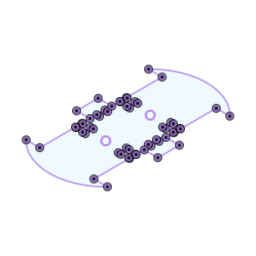
rover_M_v2_FF (Autodesk Fusion 360 design; units mm, degrees)
Autodesk Fusion 360 part; units mm, degrees
sketch "Sketch1" plane through (0, 0, 0) normal (0, 0, 1) x (1, 0, 0)
  line L0 (0, 0) -> (75, 0) construction
  line L1 (0, 0) -> (0, 145) construction
  line L2 (75, 0) -> (75, 20)
  line L3 (75, 20) -> (50, 20)
  line L4 (50, 20) -> (50, 113)
  line L5 (50, 113) -> (75, 113)
  arc A0 (75, 113) -> (0, 145) centre (0, 41.1094) ccw
  line L6 (0, 145) -> (-55.6559, 145) construction
  line L7 (-75, 0) -> (-75, 20)
  line L8 (-75, 20) -> (-50, 20)
  line L9 (-50, 20) -> (-50, 113)
  line L10 (-50, 113) -> (-75, 113)
  arc A1 (0, 145) -> (-75, 113) centre (0, 41.1094) ccw
  line L11 (75, 0) -> (75, -20)
  line L12 (75, -20) -> (50, -20)
  line L13 (50, -20) -> (50, -113)
  line L14 (50, -113) -> (75, -113)
  arc A2 (0, -145) -> (75, -113) centre (0, -41.1094) ccw
  line L15 (-50, -113) -> (-75, -113)
  line L16 (-50, -20) -> (-50, -113)
  line L17 (-75, -20) -> (-50, -20)
  line L18 (-75, 0) -> (-75, -20)
  arc A3 (-75, -113) -> (0, -145) centre (0, -41.1094) ccw
  line L19 (50, 35) -> (48.5, 35)
  line L20 (48.5, 35) -> (48.5, 47)
  line L21 (48.5, 47) -> (50, 47)
  line L22 (50, 47) -> (50, 35)
  line L23 (-50, 47) -> (-50, 35)
  line L24 (-50, 35) -> (-48.5, 35)
  line L25 (-48.5, 35) -> (-48.5, 47)
  line L26 (-48.5, 47) -> (-50, 47)
  line L27 (-48.5, -47) -> (-50, -47)
  line L28 (-50, -47) -> (-50, -35)
  line L29 (50, -47) -> (50, -35)
  line L30 (50, -35) -> (48.5, -35)
  line L31 (-50, -35) -> (-48.5, -35)
  line L32 (48.5, -35) -> (48.5, -47)
  line L33 (-48.5, -35) -> (-48.5, -47)
  line L34 (48.5, -47) -> (50, -47)
  line L35 (-50, 7.5) -> (-45, 7.5)
  line L36 (-45, 7.5) -> (-45, -7.5)
  line L37 (-45, -7.5) -> (-50, -7.5)
  line L38 (-50, -7.5) -> (-50, 7.5)
  line L39 (-45, 0) -> (0, 0) construction
  line L40 (50, 7.5) -> (45, 7.5)
  line L41 (45, 7.5) -> (45, -7.5)
  line L42 (45, -7.5) -> (50, -7.5)
  line L43 (50, -7.5) -> (50, 7.5)
  line L44 (-35.5, 48.5) -> (-30.5, 48.5)
  line L45 (-30.5, 48.5) -> (-30.5, 33.5)
  line L46 (-30.5, 33.5) -> (-35.5, 33.5)
  line L47 (-35.5, 33.5) -> (-35.5, 48.5)
  line L48 (-48.5, 41) -> (-35.5, 41) construction
  line L49 (30.5, 48.5) -> (30.5, 33.5)
  line L50 (30.5, 33.5) -> (35.5, 33.5)
  line L51 (35.5, 33.5) -> (35.5, 48.5)
  line L52 (35.5, 48.5) -> (30.5, 48.5)
  line L53 (-30.5, -48.5) -> (-30.5, -33.5)
  line L54 (-30.5, -33.5) -> (-35.5, -33.5)
  line L55 (-35.5, -33.5) -> (-35.5, -48.5)
  line L56 (-35.5, -48.5) -> (-30.5, -48.5)
  line L57 (35.5, -33.5) -> (35.5, -48.5)
  line L58 (35.5, -48.5) -> (30.5, -48.5)
  line L59 (30.5, -48.5) -> (30.5, -33.5)
  line L60 (30.5, -33.5) -> (35.5, -33.5)
  point P0 (35.5, 41)
  dimension "d6" = 75
  dimension "d7" = 145
  dimension "d8" = 20
  dimension "d9" = 25
  dimension "d10" = 93
  dimension "d11" = 15
  dimension "d12" = 1.5
  dimension "d13" = 12
  dimension "d15" = 5
  dimension "d16" = 15
  dimension "d17" = 25
  dimension "d18" = 5
  dimension "d19" = 15
  dimension "d20" = 13
  constraint coincident L0.start L1.start
  constraint horizontal L0
  constraint vertical L1
  constraint perpendicular L0 L2
  constraint perpendicular L2 L3
  constraint perpendicular L3 L4
  constraint perpendicular L4 L5
  constraint equal L3 L5
  constraint perpendicular L1 L6
  constraint tangent A0 L6
  constraint symmetric L0.end L1 L7.start
  constraint symmetric A0.end L1 L6.start
  constraint symmetric L1 L2.end L7.end
  constraint symmetric L1 L3.end L8.end
  constraint symmetric L1 L4.end L9.end
  constraint symmetric L1 L5.end L10.end
  constraint symmetric L1 A0 A1
  constraint symmetric L2.start L0 L11.start
  constraint symmetric L0 L1.end A2.start
  constraint symmetric L0 L2.end L11.end
  constraint symmetric L0 L3.end L12.end
  constraint symmetric L0 L4.end L13.end
  constraint symmetric L0 L5.end L14.end
  constraint symmetric L0 A0 A2
  constraint symmetric L0 L7.start L18.start
  constraint symmetric L0 L7.end L17.start
  constraint symmetric L0 L8.end L16.start
  constraint symmetric L0 L9.end L15.start
  constraint symmetric L0 L10.end L15.end
  constraint symmetric L0 A1 A3
  constraint horizontal L19
  constraint vertical L20
  constraint horizontal L21
  constraint vertical L22
  constraint coincident L4 L19.start
  constraint symmetric L1 L19.start L23.end
  constraint symmetric L1 L19.end L24.end
  constraint symmetric L1 L20.end L25.end
  constraint symmetric L1 L21.end L23.start
  constraint symmetric L0 L19.start L29.end
  constraint symmetric L0 L19.end L30.end
  constraint symmetric L0 L20.end L32.end
  constraint symmetric L0 L21.end L29.start
  constraint symmetric L0 L23.start L27.end
  constraint symmetric L0 L23.end L28.end
  constraint symmetric L0 L24.end L31.end
  constraint symmetric L0 L25.end L27.start
  constraint horizontal L35
  constraint vertical L36
  constraint horizontal L37
  constraint vertical L38
  constraint midpoint L36 L39.start
  constraint horizontal L39
  constraint symmetric L1 L35.start L40.start
  constraint symmetric L1 L35.end L40.end
  constraint symmetric L1 L36.end L41.end
  constraint symmetric L1 L37.end L42.end
  constraint horizontal L44
  constraint vertical L45
  constraint horizontal L46
  constraint vertical L47
  constraint midpoint L25 L48.start
  constraint perpendicular L47 L48
  constraint midpoint L47 L48.end
  constraint symmetric L1 L44.start L51.end
  constraint symmetric L1 L44.end L49.start
  constraint symmetric L1 L45.end L49.end
  constraint symmetric L1 L46.end L50.end
  constraint symmetric L1 L48.end P0
  constraint symmetric L39 L44.start L55.end
  constraint symmetric L39 L44.end L53.start
  constraint symmetric L39 L45.end L53.end
  constraint symmetric L39 L46.end L54.end
  constraint symmetric L0 L49.start L58.end
  constraint symmetric L0 L49.end L59.end
  constraint symmetric L0 L50.end L57.start
  constraint symmetric L0 L51.end L57.end
  measures "d6" distance of L0.start L0.end
  measures "d7" distance of L0.start L1.end
  measures "d8" distance of L0.end L2.end
  measures "d9" distance of L2.end L3.end
  measures "d10" distance of L3.end L4.end
  measures "d11" distance of L3 L19
  measures "d12" distance of L19.start L19.end
  measures "d13" distance of L19.end L20.end
  measures "d15" distance of L35.start L35.end
  measures "d16" distance of L35.start L37.end
  measures "d17" distance of L7.start L38
  measures "d18" distance of L44.start L44.end
  measures "d19" distance of L44.start L46.end
  measures "d20" distance of L48.start L48.end
extrude "Extrude1" add sketch "Sketch1" along normal blind 3 contours L2 L3 L4 L5 A0 L7 L8 L9 L10 A1 L11 L12 L13 L14 A2 L15 L16 L17 L18 A3 L19 L20 L21 L24 L25 L26 L27 L30 L31 L32 L33 L34
sketch "Sketch2" plane through (0, 0, 3) normal (0, 0, 1) x (-1, 0, 0)
  line L0 (-30.5, 48.5) -> (-30.5, 33.5)
  line L1 (-30.5, 33.5) -> (-35.5, 33.5)
  line L2 (-35.5, 33.5) -> (-35.5, 48.5)
  line L3 (-35.5, 48.5) -> (-30.5, 48.5)
  line L4 (45, 7.5) -> (50, 7.5)
  line L5 (50, 7.5) -> (50, -7.5)
  line L6 (50, -7.5) -> (45, -7.5)
  line L7 (45, -7.5) -> (45, 7.5)
  line L8 (30.5, 48.5) -> (35.5, 48.5)
  line L9 (35.5, 48.5) -> (35.5, 33.5)
  line L10 (35.5, 33.5) -> (30.5, 33.5)
  line L11 (30.5, 33.5) -> (30.5, 48.5)
  line L12 (-30.5, -48.5) -> (-35.5, -48.5)
  line L13 (-35.5, -48.5) -> (-35.5, -33.5)
  line L14 (-35.5, -33.5) -> (-30.5, -33.5)
  line L15 (-30.5, -33.5) -> (-30.5, -48.5)
  line L16 (30.5, -33.5) -> (35.5, -33.5)
  line L17 (35.5, -33.5) -> (35.5, -48.5)
  line L18 (35.5, -48.5) -> (30.5, -48.5)
  line L19 (30.5, -48.5) -> (30.5, -33.5)
  line L20 (-50, -7.5) -> (-50, 7.5)
  line L21 (-50, 7.5) -> (-45, 7.5)
  line L22 (-45, 7.5) -> (-45, -7.5)
  line L23 (-45, -7.5) -> (-50, -7.5)
  line L24 (-75, 20) -> (-75, -20)
  line L25 (-75, -20) -> (-50, -20)
  line L26 (-50, -20) -> (-50, -35)
  line L27 (-50, -35) -> (-48.5, -35)
  line L28 (-48.5, -35) -> (-48.5, -47)
  line L29 (-48.5, -47) -> (-50, -47)
  line L30 (-50, -47) -> (-50, -113)
  line L31 (-50, -113) -> (-75, -113)
  arc A0 (-75, -113) -> (75, -113) centre (0, -41.1094) ccw
  line L32 (75, -113) -> (50, -113)
  line L33 (50, -113) -> (50, -47)
  line L34 (50, -47) -> (48.5, -47)
  line L35 (48.5, -47) -> (48.5, -35)
  line L36 (48.5, -35) -> (50, -35)
  line L37 (50, -35) -> (50, -20)
  line L38 (50, -20) -> (75, -20)
  line L39 (75, -20) -> (75, 20)
  line L40 (75, 20) -> (50, 20)
  line L41 (50, 20) -> (50, 35)
  line L42 (50, 35) -> (48.5, 35)
  line L43 (48.5, 35) -> (48.5, 47)
  line L44 (48.5, 47) -> (50, 47)
  line L45 (50, 47) -> (50, 113)
  line L46 (50, 113) -> (75, 113)
  arc A1 (75, 113) -> (-75, 113) centre (0, 41.1094) ccw
  line L47 (-75, 113) -> (-50, 113)
  line L48 (-50, 113) -> (-50, 47)
  line L49 (-50, 47) -> (-48.5, 47)
  line L50 (-48.5, 47) -> (-48.5, 35)
  line L51 (-48.5, 35) -> (-50, 35)
  line L52 (-50, 35) -> (-50, 20)
  line L53 (-50, 20) -> (-75, 20)
equation "d6 = ( 150 / 2 ) * 1 mm"
equation "d7 = ( 290 / 2 ) * 1 mm"
equation "d8 = ( 40 / 2 ) * 1 mm"
